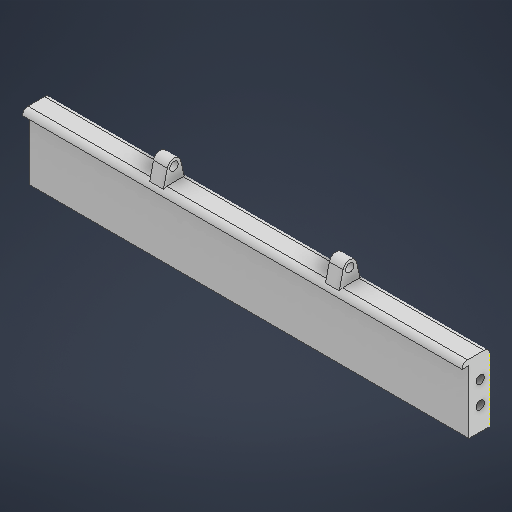
# Autodesk Inventor part: plate
Saved by Autodesk Inventor 2027 (Build 310192000, 192)
## iProperties
Created: 2026-07-09
Part Number: plate
Material: Generic
Document SubType Name: Modeling
Designer: uchiha
Density: 1 g/cm^3
Appearance: Default
Author: uchiha
Autodesk Inventor part; units mm, degrees
sketch "Sketch1" plane through (0, 0, 0) normal (0, 0, 1) x (1, 0, 0)
  line L0 (40, 12.5) -> (-40, 12.5)
  line L1 (-40, 12.5) -> (-40, -12.5)
  line L2 (-40, -12.5) -> (40, -12.5)
  line L3 (40, -12.5) -> (40, 12.5)
  line L4 (40, 12.5) -> (-40, -12.5) construction
  line L5 (-40, 12.5) -> (40, -12.5) construction
  point P0 (0, 0)
  dimension "d0" = 80
  dimension "d1" = 25
  constraints: 12 end point, 2 midpoint, 2 parallel, 1 horizontal, 1 perpendicular
  measures "d0" distance of L0.start L0.end
  measures "d1" distance of L2.end L0.start
extrude "Extrusion1" add sketch "Sketch1" along normal blind 10
ref_plane "Work Plane1" through (-8, -12.5, 0) normal (1, 0, 0) x (0, 0, -1)
sketch "Sketch2" plane through (-8, -12.5, 0) normal (1, 0, 0) x (0, 0, -1)
  circle A0 centre (-5.3658, 30) radius 2.5
  line L0 (0, 25) -> (-10, 25) projected
  line L1 (-9.1092, 25) -> (-7.7995, 30.572)
  line L2 (-2.9321, 30.572) -> (-1.6224, 25)
  point P0 (0, 12.5)
  dimension "d5" = 5
  dimension "d11" = 5
  constraints: 4 end point, 2 point on circle, 2 point on line, 2 tangent, 1 centre point, 1 equal length
  measures "d5" diameter of A0
  measures "d11" distance from line of L0 A0.centre
extrude "Extrusion2" add sketch "Sketch2" along normal mid plane 5
sketch "Sketch3" plane through (-5.5, -12.5, 0) normal (1, 0, 0) x (0, 0, -1)
  arc A0 (-2.9321, 30.572) -> (-7.7995, 30.572) centre (-5.3658, 30) ccw projected
  circle A1 centre (-5.3658, 30) radius 1.5
  point P0 (0, 12.5)
  dimension "d8" = 3
  constraints: 1 centre point, 1 coincident
  measures "d8" diameter of A1
extrude "Extrusion3" cut sketch "Sketch3" against normal blind 20
sketch "Sketch4" plane through (0, 0, 0) normal (0, 0, -1) x (-1, 0, 0)
  point P0 (0, 0)
sketch "Sketch5" plane through (-40, -12.5, 0) normal (-1, 0, 0) x (0, 0, 1)
  point P0 (0, 12.5)
ref_plane "Work Plane2" through (-40, -12.5, 0) normal (-1, 0, 0) x (0, 0, 1)
mirror "Mirror1" about plane through (-40, 12.5, 0) normal (-1, 0, 0) of "Extrusion2", "Extrusion1"
fillet "Fillet1" radius 2 2 edges at (-40, 12.5, 10) (-40, 12.5, 0)
sketch "Sketch6" plane through (-74.5, 17.5, 5.3658) normal (-1, 0, 0) x (0, 0, 1)
  circle A0 centre (0, 0) radius 1.5
  point P0 (-5.3658, -17.5)
  constraints: 1 centre point
extrude "Extrusion4" cut sketch "Sketch6" against normal blind 20
ref_plane "Work Plane3" through (20, 10.5, 6) normal (0, 0, -1) x (-1, 0, 0)
sketch "Sketch7" plane through (40, -12.5, 10) normal (1, 0, 0) x (0, 0, -1)
  circle A0 centre (6.606, 16.5) radius 1.5
  circle A1 centre (6.606, 8.5) radius 1.5
  line L0 (10, 0) -> (0, 0) projected
  line L1 (10, 0) -> (10, 23) projected
  point P0 (10, 12.5)
  point P1 (5, 0)
  dimension "d16" = 3
  dimension "d17" = 3
  dimension "d19" = 8.5
  dimension "d20" = 8
  dimension "d32" = 3.394
  dimension "d33" = 3.394
  constraints: 2 centre point, 1 midpoint
  measures "d16" diameter of A0
  measures "d17" diameter of A1
  measures "d19" vertical distance of point (5, 0) A1.centre
  measures "d20" distance of A0.centre A1.centre
  measures "d32" distance from line of L1 A0.centre
  measures "d33" distance from line of L1 A1.centre
extrude "Extrusion5" cut sketch "Sketch7" against normal blind 8
ref_plane "Work Plane4" through (-120, -12.5, 0) normal (-1, 0, 0) x (0, 0, 1)
mirror "Mirror2" about plane through (-40, -12.5, 0) normal (-1, 0, 0) of "Extrusion5"
thread "Thread1" size "M3x0.5" class "6H" standard "ANSI Metric M Profile" length 10
thread "Thread2" size "M3x0.5" class "6H" standard "ANSI Metric M Profile" length 10
thread "Thread3" size "M3x0.5" class "6H" standard "ANSI Metric M Profile" length 10
thread "Thread4" size "M3x0.5" class "6H" standard "ANSI Metric M Profile" length 10
sketch "Sketch8" plane through (0, 0, 0) normal (0, 0, -1) x (-1, 0, 0)
  line L0 (-40, 10.5) -> (120, 10.5) construction
  line L1 (-40, -12.5) -> (-40, 10.5) construction
  line L2 (-40, -12.5) -> (120, -12.5) construction
  line L3 (120, -12.5) -> (120, 10.5) projected
  point P0 (0, 0)
sketch "Sketch9" plane through (0, 0, 10) normal (0, 0, 1) x (1, 0, 0)
  line L0 (-120, 10.5) -> (40, 10.5) projected
  line L1 (-120, -12.5) -> (-120, 10.5) projected
  line L2 (40, -12.5) -> (-120, -12.5) projected
  line L3 (40, -12.5) -> (40, 10.5) projected
  point P0 (0, 0)
extrude "Extrusion6" cut sketch "Sketch9" against normal blind 2.5
body "Solid1"
